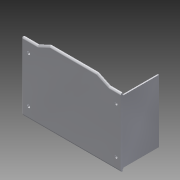
# Autodesk Inventor part: Simple3DPrintBackplate01
Saved by Autodesk Inventor 2015 (Build 190159000, 159)
## iProperties
Created: 2015-09-24
Part Number: Simple3DPrintBackplate01
Material: Aluminum 6061 Black Anodized
Document SubType Name: Modeling
Designer: -
Density: 2.71 g/cm^3
Appearance: Aluminum - Flat
Author: -
Autodesk Inventor part; units mm, degrees
ref_plane "YZ Plane" through (0, 0, 0) normal (1, 0, 0) x (0, 1, 0)
ref_plane "XZ Plane" through (0, 0, 0) normal (0, 1, 0) x (-1, 0, 0)
ref_plane "XY Plane" through (0, 0, 0) normal (0, 0, 1) x (1, 0, 0)
sketch "Sketch1" plane through (0, 0, 0) normal (0, 0, 1) x (1, 0, 0)
  line L0 (25.0566, 47.4388) -> (-25.0566, 47.4388)
  line L1 (-25.9018, 47.2514) -> (-38.0982, 41.5642)
  line L2 (-38.9434, 41.3768) -> (-53.924, 41.3768)
  line L3 (-55.924, 39.3768) -> (-55.924, -30.1412)
  line L4 (-53.924, -32.1412) -> (62.994, -32.1412)
  line L5 (64.994, -30.1412) -> (64.994, 39.3768)
  line L6 (62.994, 41.3768) -> (38.9434, 41.3768)
  line L7 (38.0982, 41.5642) -> (25.9018, 47.2514)
  line L8 (0, 0) -> (0, 61.2972) construction
  arc A0 (64.994, 39.3768) -> (62.994, 41.3768) centre (62.994, 39.3768) ccw
  arc A1 (62.994, -32.1412) -> (64.994, -30.1412) centre (62.994, -30.1412) ccw
  arc A2 (-55.924, -30.1412) -> (-53.924, -32.1412) centre (-53.924, -30.1412) ccw
  arc A3 (-53.924, 41.3768) -> (-55.924, 39.3768) centre (-53.924, 39.3768) ccw
  arc A4 (-38.9434, 41.3768) -> (-38.0982, 41.5642) centre (-38.9434, 43.3768) ccw
  arc A5 (-25.0566, 47.4388) -> (-25.9018, 47.2514) centre (-25.0566, 45.4388) ccw
  arc A6 (25.9018, 47.2514) -> (25.0566, 47.4388) centre (25.0566, 45.4388) ccw
  arc A7 (38.0982, 41.5642) -> (38.9434, 41.3768) centre (38.9434, 43.3768) ccw
  point P0 (25.5, 47.4388)
  point P1 (-25.5, 47.4388)
  point P2 (-38.5, 41.3768)
  point P3 (-55.924, 41.3768)
  point P4 (-55.924, -32.1412)
  point P5 (64.994, 41.3768)
  point P6 (38.5, 41.3768)
  point P7 (0, 47.4388)
  dimension "d48" = 51
  dimension "d50" = 155
  dimension "d51" = 155
  dimension "d52" = 13
  dimension "d53" = 17.424
  dimension "d54" = 26.494
  dimension "d55" = 73.518
  dimension "d56" = 13
  dimension "d57" = 2
  constraints: 18 end point, 16 point on circle, 16 point on line, 16 tangent, 8 centre point, 7 equal radius, 4 perpendicular, 2 horizontal, 1 midpoint, 1 parallel, 1 vertical, 1 other
  measures "d48" distance of point (25.5, 47.439) point (-25.5, 47.439)
  measures "d50" angle of L0 L7
  measures "d51" angle of L0 L1
  measures "d52" horizontal distance of point (-38.5, 41.377) point (-25.5, 47.439)
  measures "d53" distance of point (-38.5, 41.377) point (-55.924, 41.377)
  measures "d54" distance of point (64.994, 41.377) point (38.5, 41.377)
  measures "d55" distance of point (-55.924, 41.377) point (-55.924, -32.141)
  measures "d56" horizontal distance of point (25.5, 47.439) point (38.5, 41.377)
  measures "d57" radius of A0
extrude "Extrusion1" add sketch "Sketch1" along normal blind 2
chamfer "Chamfer1" distance 1.5 distance2 1 16 edges at (50.9687, 41.3768, 2) (38.5105, 41.4242, 2) (32, 44.4078, 2) (25.4895, 47.3914, 2) (0, 47.4388, 2) (-25.4895, 47.3914, 2) (-32, 44.4078, 2) (-38.5105, 41.4242, 2) (-46.4337, 41.3768, 2) (-55.3382, 40.791, 2) (-55.924, 4.6178, 2) (-55.3382, -31.5554, 2) (4.535, -32.1412, 2) (64.4082, -31.5554, 2) (64.994, 4.6178, 2) (64.4082, 40.791, 2) measured on face at (11.3755, -5.6145, 2)
fillet "Fillet1" radius 2 16 edges at (-54.2776, 39.7304, 2) (-46.4337, 39.8768, 2) (-38.1859, 39.9598, 2) (-31.3661, 43.0484, 2) (-25.1648, 45.927, 2) (0, 45.9388, 2) (25.1648, 45.927, 2) (31.3661, 43.0484, 2) (38.1859, 39.9598, 2) (50.9687, 39.8768, 2) (63.3476, 39.7304, 2) (63.494, 4.6178, 2) (63.3476, -30.4947, 2) (4.535, -30.6412, 2) (-54.2776, -30.4947, 2) (-54.424, 4.6178, 2)
fillet "Fillet2" radius 1 16 edges at (-55.3382, -31.5554, 1) (4.535, -32.1412, 1) (64.4082, -31.5554, 1) (64.994, 4.6178, 1) (64.4082, 40.791, 1) (50.9687, 41.3768, 1) (38.5105, 41.4242, 1) (32, 44.4078, 1) (25.4895, 47.3914, 1) (0, 47.4388, 1) (-25.4895, 47.3914, 1) (-32, 44.4078, 1) (-38.5105, 41.4242, 1) (-46.4337, 41.3768, 1) (-55.3382, 40.791, 1) (-55.924, 4.6178, 1)
feature "Lip1" [suppressed]
sketch "Sketch8" plane through (0, 0, 0) normal (0, 0, -1) x (-1, 0, 0)
  line L0 (-64.994, 39.3768) -> (-64.994, -30.1412) projected
  arc A0 (-64.994, -30.1412) -> (-62.994, -32.1412) centre (-62.994, -30.1412) ccw projected
  line L1 (-62.994, -32.1412) -> (53.924, -32.1412) projected
  arc A1 (53.924, -32.1412) -> (55.924, -30.1412) centre (53.924, -30.1412) ccw projected
  line L2 (55.924, -30.1412) -> (55.924, 39.3768) projected
  arc A2 (55.924, 39.3768) -> (53.924, 41.3768) centre (53.924, 39.3768) ccw projected
  line L3 (53.924, 41.3768) -> (38.9434, 41.3768) projected
  arc A3 (38.0982, 41.5642) -> (38.9434, 41.3768) centre (38.9434, 43.3768) ccw projected
  line L4 (38.0982, 41.5642) -> (25.9018, 47.2514) projected
  arc A4 (25.9018, 47.2514) -> (25.0566, 47.4388) centre (25.0566, 45.4388) ccw projected
  line L5 (25.0566, 47.4388) -> (-25.0566, 47.4388) projected
  arc A5 (-25.0566, 47.4388) -> (-25.9018, 47.2514) centre (-25.0566, 45.4388) ccw projected
  line L6 (-25.9018, 47.2514) -> (-38.0982, 41.5642) projected
  arc A6 (-38.9434, 41.3768) -> (-38.0982, 41.5642) centre (-38.9434, 43.3768) ccw projected
  line L7 (-38.9434, 41.3768) -> (-62.994, 41.3768) projected
  arc A7 (-62.994, 41.3768) -> (-64.994, 39.3768) centre (-62.994, 39.3768) ccw projected
  line L8 (-60.894, 39.2768) -> (-38.9434, 39.2768)
  arc A8 (-38.9434, 39.2768) -> (-37.2107, 39.661) centre (-38.9434, 43.3768) ccw
  line L9 (-37.2107, 39.661) -> (-25.8381, 44.964)
  line L10 (-24.1477, 45.3388) -> (24.1477, 45.3388)
  line L11 (25.8381, 44.964) -> (37.2107, 39.661)
  arc A9 (37.2107, 39.661) -> (38.9434, 39.2768) centre (38.9434, 43.3768) ccw
  line L12 (38.9434, 39.2768) -> (51.824, 39.2768)
  line L13 (53.824, 37.2768) -> (53.824, -28.0412)
  line L14 (51.824, -30.0412) -> (-60.894, -30.0412)
  line L15 (-62.894, -28.0412) -> (-62.894, 37.2768)
  arc A10 (-60.894, 39.2768) -> (-62.894, 37.2768) centre (-60.894, 37.2768) ccw
  arc A11 (-62.894, -28.0412) -> (-60.894, -30.0412) centre (-60.894, -28.0412) ccw
  arc A12 (51.824, -30.0412) -> (53.824, -28.0412) centre (51.824, -28.0412) ccw
  arc A13 (53.824, 37.2768) -> (51.824, 39.2768) centre (51.824, 37.2768) ccw
  arc A14 (-24.1477, 45.3388) -> (-25.8381, 44.964) centre (-24.1477, 41.3388) ccw
  arc A15 (25.8381, 44.964) -> (24.1477, 45.3388) centre (24.1477, 41.3388) ccw
  point P0 (0, 0)
  dimension "d62" = 2.1
  dimension "d63" = 2
  dimension "d64" = 4
  constraints: 16 end point, 16 point on circle, 12 tangent, 8 centre point, 4 equal radius, 9 other
  measures "d62" distance between parallel lines of L7 L8
  measures "d63" radius of A10
  measures "d64" radius of A14
extrude "Extrusion7" add sketch "Sketch8" along normal blind 1 contours L8 A8 L9 A14 L10 A15 L11 A9 L12 A13 L13 A12 L14 A11 L15 A10
sketch "Sketch4" plane through (0, 0, 2) normal (0, 0, 1) x (1, 0, 0)
  line L0 (92.6097, 61.0907) -> (51.0597, 61.0907)
  line L1 (51.0597, 61.0907) -> (51.0597, -62.6292)
  line L2 (51.0597, -62.6292) -> (92.6097, -62.6292)
  line L3 (92.6097, -62.6292) -> (92.6097, 61.0907)
  line L4 (64.5487, 39.3768) -> (64.5487, -30.1412) projected
  point P0 (0, 0)
  dimension "d21" = 123.7199
  dimension "d22" = 41.55
  dimension "d58" = 13.489
  constraints: 8 end point, 2 parallel, 1 horizontal, 1 perpendicular
  measures "d21" distance between parallel lines of L2 L0
  measures "d22" distance between parallel lines of L3 L1
  measures "d58" distance between parallel lines of L1 L4
extrude "Extrusion3" cut sketch "Sketch4" against normal blind 10
sketch "Sketch7" plane through (0, 0, 0) normal (0, 0, -1) x (-1, 0, 0)
  line L0 (-51.0597, 38.2572) -> (-49.7257, 38.2572)
  line L1 (-49.7257, 38.2572) -> (-49.7257, -29.0608)
  line L2 (-49.7257, -29.0608) -> (-51.0597, -29.0608)
  line L3 (-51.0597, -29.0608) -> (-51.0597, 38.2572)
  line L4 (-51.0597, -30.0412) -> (-51.0597, -32.1412) projected
  line L5 (53.924, -30.8108) -> (-51.0597, -30.8108) projected
  line L6 (-51.0597, 42.7072) -> (-38.8527, 42.7072) projected
  point P0 (0, 0)
  point P1 (-51.0597, -28.8108)
  point P2 (-51.0597, 40.7072)
  point P3 (-32.4217, 42.6092)
  dimension "d35" = 1.334
  dimension "d59" = 1.75
  dimension "d60" = 4.45
  dimension "d61" = 67.318
  constraints: 8 end point, 2 parallel, 1 horizontal, 1 perpendicular, 1 vertical, 1 other
  measures "d35" distance between parallel lines of L3 L1
  measures "d59" distance between parallel lines of L5 L2
  measures "d60" distance between parallel lines of L0 L6
  measures "d61" distance between parallel lines of L2 L0
extrude "Extrusion6" add sketch "Sketch7" along normal blind 39
sketch "Sketch9" plane through (0, 0, 2) normal (0, 0, 1) x (1, 0, 0)
  circle A0 centre (-47.914, 29.3988) radius 1.5 projected
  circle A1 centre (-47.914, -20.1312) radius 1.5 projected
  circle A2 centre (46.066, 29.3988) radius 1.5 projected
  circle A3 centre (46.066, -20.1312) radius 1.5 projected
  point P0 (0, 0)
extrude "Extrusion8" cut sketch "Sketch9" against normal blind 10
body "Solid1"
